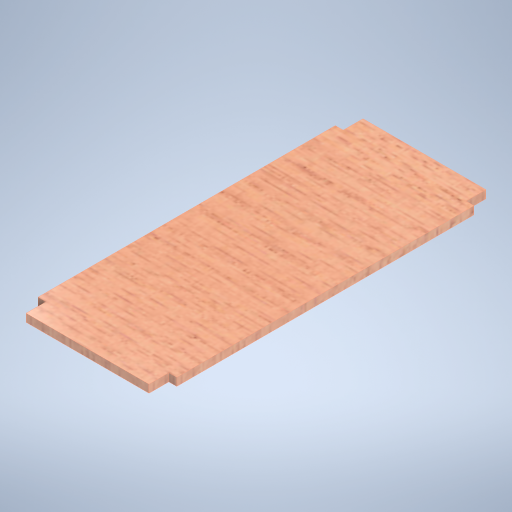
# Autodesk Inventor part: ER_lipo_sikiri_up
Saved by Autodesk Inventor 2023 (Build 270158000, 158)
## iProperties
Created: 2023-03-05
Part Number: ER_lipo_sikiri_up
Material: 木材 (オーク)
Document SubType Name: Modeling
Designer: mkhr7
Density: 0.76 g/cm^3
Appearance: ホワイト オーク材 - ナチュラル 標準の光沢
Author: mkhr7
Autodesk Inventor part; units mm, degrees
ref_plane "YZ Plane" through (0, 0, 0) normal (1, 0, 0) x (0, 1, 0)
ref_plane "XZ Plane" through (0, 0, 0) normal (0, 1, 0) x (-1, 0, 0)
ref_plane "XY Plane" through (0, 0, 0) normal (0, 0, 1) x (1, 0, 0)
sketch "スケッチ1" plane through (0, 0, 0) normal (0, 1, 0) x (-1, 0, 0)
  line L0 (0, 0) -> (62, 0)
  line L1 (62, 0) -> (62, -170)
  line L2 (62, -170) -> (0, -170)
  line L3 (0, -170) -> (0, 0)
  line L4 (62, -10) -> (66, -10)
  line L5 (66, -10) -> (66, -160)
  line L6 (66, -160) -> (62, -160)
  line L7 (62, -160) -> (62, -10)
  line L8 (0, -10) -> (-4, -10)
  line L9 (-4, -10) -> (-4, -160)
  line L10 (-4, -160) -> (0, -160)
  line L11 (0, -160) -> (0, -10)
  point P0 (0, -160)
  dimension "d0" = 62
  dimension "d1" = 170
  dimension "d2" = 4
  dimension "d3" = 150
  dimension "d4" = 4
  dimension "d5" = 150
  dimension "d6" = 10
  dimension "d7" = 10
  constraints: 24 end point, 6 parallel, 3 horizontal, 3 perpendicular, 2 point on line
  measures "d0" distance of L1.end L2.end
  measures "d1" distance of L0.end L1.end
  measures "d2" distance of L5.end L6.end
  measures "d3" distance of L4.end L5.end
  measures "d4" distance of L10.end L9.end
  measures "d5" distance of L9.end L8.end
  measures "d6" distance between parallel lines of L0 L4
  measures "d7" distance between parallel lines of L0 L8
extrude "押し出し1" add sketch "スケッチ1" along normal blind 4
